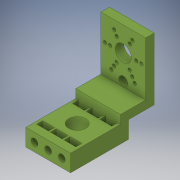
# Autodesk Inventor part: 000.406 - Проставка
Saved by Autodesk Inventor 2019 (Build 230136000, 136)
## iProperties
Created: 2020-02-29
Part Number: 000.406 - Проставка
Material: Пластик АБС
Document SubType Name: Modeling
Designer: Петров Иван
Density: 1.06 g/cm^3
Appearance: Оливково-зеленый
Author: Петров Иван
Autodesk Inventor part; units mm, degrees
ref_plane "YZ Plane" through (0, 0, 0) normal (1, 0, 0) x (0, 1, 0)
ref_plane "XZ Plane" through (0, 0, 0) normal (0, 1, 0) x (-1, 0, 0)
ref_plane "XY Plane" through (0, 0, 0) normal (0, 0, 1) x (1, 0, 0)
sketch "Эскиз1" plane through (0, 0, 0) normal (0, 1, 0) x (-1, 0, 0)
  line L0 (-13.1, 17) -> (13.1, 17)
  line L1 (13.1, 17) -> (13.1, -17)
  line L2 (13.1, -17) -> (-13.1, -17)
  line L3 (-13.1, -17) -> (-13.1, 17)
  line L4 (-13.1, 17) -> (13.1, -17) construction
  line L5 (13.1, 17) -> (-13.1, -17) construction
  point P0 (0, 0)
  dimension "d0" = 26.2
  dimension "d1" = 34
  constraints: 12 end point, 2 midpoint, 2 parallel, 1 horizontal, 1 perpendicular
  measures "d0" distance of L1.end L2.end
  measures "d1" distance of L0.end L1.end
extrude "Выдавливание1" add sketch "Эскиз1" along normal blind 10
sketch "Эскиз2" plane through (-13.1, 0, 17) normal (0, 0, 1) x (1, 0, 0)
  line L0 (0, 10) -> (26.2, 10) projected
  line L1 (13.1, 10) -> (13.1, 5)
  circle A0 centre (13.1, 5) radius 2
  point P0 (13.1, 0)
  dimension "d4" = 5
  dimension "d5" = 4
  constraints: 2 end point, 1 centre point, 1 coincident, 1 midpoint, 1 vertical
  measures "d4" distance of L1.start L1.end
  measures "d5" diameter of A0
extrude "Выдавливание2" cut sketch "Эскиз2" against normal blind 10
sketch "Эскиз4" plane through (0, 10, 0) normal (0, 1, 0) x (1, 0, 0)
  line L0 (2, -7) -> (-2, -7) projected
  line L1 (3.4971, -12.25) -> (-3.4971, -12.25)
  line L2 (-3.4971, -12.25) -> (-3.4971, -8.75)
  line L3 (-3.4971, -8.75) -> (3.4971, -8.75)
  line L4 (3.4971, -8.75) -> (3.4971, -12.25)
  line L5 (3.4971, -12.25) -> (-3.4971, -8.75) construction
  line L6 (-3.4971, -12.25) -> (3.4971, -8.75) construction
  point P0 (0, 0)
  point P1 (0, -10.5)
  dimension "d55" = 10.5
  constraints: 12 end point, 2 midpoint, 2 parallel, 1 perpendicular
  measures "d55" distance of point (0, 0) point (0, -10.5)
extrude "Выдавливание3" cut sketch "Эскиз4" against normal through all
pattern_linear "Прямоуг.массив2" count 3 spacing 8 along (1, 0, 0) of "Выдавливание2", "Выдавливание3" first direction both ways yes
mirror "Зеркальное отражение2" about plane through (0, 0, 0) normal (0, 0, 1) of "Выдавливание2", "Выдавливание3", "Прямоуг.массив2"
sketch "Эскиз5" plane through (0, 10, 0) normal (0, 1, 0) x (1, 0, 0)
  line L0 (-13.1, -17) -> (-13.1, 17) projected
  line L1 (13.1, 17) -> (13.1, -17) projected
  line L2 (-13.1, 17) -> (13.1, 17)
  line L3 (13.1, 17) -> (13.1, 12.25)
  line L4 (13.1, 12.25) -> (-13.1, 12.25)
  line L5 (-13.1, 12.25) -> (-13.1, 17)
  line L6 (-2, 12.25) -> (2, 12.25) projected
  point P0 (0, 0)
  dimension "d17" = 0
  constraints: 8 end point, 2 parallel, 1 horizontal, 1 perpendicular, 1 point on line
  measures "d17" distance between parallel lines of L6 L4
extrude "Выдавливание4" add sketch "Эскиз5" along normal blind 5
sketch "Эскиз7" plane through (13.1, 0, -17) normal (0, 0, -1) x (-1, 0, 0)
  line L0 (26.2, 0) -> (26.2, 15) projected
  line L1 (26.2, 10) -> (0, 10) projected
  line L2 (26.2, 15) -> (0, 15)
  line L3 (0, 15) -> (0, 10)
  line L4 (0, 10) -> (26.2, 10)
  line L5 (26.2, 10) -> (26.2, 15)
  point P0 (13.1, 0)
  constraints: 8 end point, 2 parallel, 1 horizontal, 1 perpendicular
extrude "Выдавливание6" add sketch "Эскиз7" along normal blind 15
sketch "Эскиз8" plane through (0, 15, 0) normal (0, 1, 0) x (1, 0, 0)
  line L0 (-13.1, 32) -> (13.1, 32)
  line L1 (13.1, 32) -> (13.1, 27)
  line L2 (13.1, 27) -> (-13.1, 27)
  line L3 (-13.1, 27) -> (-13.1, 32)
  line L4 (-13.1, 32) -> (13.1, 32) projected
  point P0 (0, 0)
  point P1 (-13.1, 17)
  dimension "d33" = 5
  dimension "d37" = 0
  constraints: 8 end point, 2 parallel, 1 horizontal, 1 perpendicular
  measures "d33" distance of L0.end L1.end
  measures "d37" distance between parallel lines of L4 L0
extrude "Выдавливание7" add sketch "Эскиз8" along normal blind 31.5
sketch "Эскиз10" plane through (-13.1, 15, -27) normal (0, 0, 1) x (1, 0, 0)
  line L0 (0, 0) -> (26.2, 0) projected
  arc A0 (4.1835, 6.1603) -> (7.4622, 3.7057) centre (6.1878, 5.4205) ccw
  line L1 (7.4622, 3.7057) -> (12.988, 10.2609)
  line L2 (12.988, 10.2609) -> (18.2196, 3.9682)
  arc A1 (18.2196, 3.9682) -> (21.9847, 5.5803) centre (19.8625, 5.334) ccw
  line L3 (21.9847, 5.5803) -> (19.0707, 13.6434)
  line L4 (19.0707, 13.6434) -> (27.1362, 15.0277)
  arc A2 (27.1362, 15.0277) -> (27.6225, 19.0945) centre (26.7747, 17.1334) ccw
  line L5 (27.6225, 19.0945) -> (19.1827, 20.6024)
  line L6 (19.1827, 20.6024) -> (22.0165, 28.2795)
  arc A3 (22.0165, 28.2795) -> (18.7378, 30.7341) centre (20.0122, 29.0193) ccw
  line L7 (18.7378, 30.7341) -> (13.212, 24.1789)
  line L8 (13.212, 24.1789) -> (7.9804, 30.4716)
  arc A4 (7.9804, 30.4716) -> (4.2153, 28.8595) centre (6.3375, 29.1058) ccw
  line L9 (4.2153, 28.8595) -> (7.1293, 20.7964)
  line L10 (7.1293, 20.7964) -> (-0.9362, 19.412)
  arc A5 (-0.9362, 19.412) -> (-1.4225, 15.3453) centre (-0.5747, 17.3063) ccw
  line L11 (-1.4225, 15.3453) -> (7.0173, 13.8374)
  line L12 (7.0173, 13.8374) -> (4.1835, 6.1603)
  circle A6 centre (9.2206, 10.5975) radius 1
  circle A7 centre (6.1878, 5.4205) radius 1
  circle A8 centre (2.4252, 17.2874) radius 1
  circle A9 centre (9.3046, 23.8908) radius 1
  circle A10 centre (6.3375, 29.1058) radius 1
  circle A11 centre (18.4958, 26.4308) radius 1
  circle A12 centre (20.7748, 17.1714) radius 1
  circle A13 centre (26.7747, 17.1334) radius 1
  circle A14 centre (18.3789, 7.9415) radius 1
  circle A15 centre (13.1, 17.2199) radius 4.75
  circle A16 centre (19.8625, 5.334) radius 1
  circle A17 centre (16.8954, 10.549) radius 1
  circle A18 centre (23.7748, 17.1524) radius 1
  circle A19 centre (20.0122, 29.0193) radius 1
  circle A20 centre (16.9794, 23.8422) radius 1
  circle A21 centre (7.8211, 26.4983) radius 1
  circle A22 centre (-0.5747, 17.3063) radius 1
  circle A23 centre (5.4252, 17.2684) radius 1
  circle A24 centre (7.7042, 8.009) radius 1
  circle A25 centre (13.1, 17.2199) radius 1.875
  point P0 (13.1, -15)
  dimension "d41" = 6.9599
  dimension "d42" = 6.9599
  dimension "d43" = 6.959
  dimension "d44" = 6.959
  dimension "d45" = 6.9599
  dimension "d46" = 6.9599
  dimension "d47" = 3
  constraints: 26 centre point, 24 end point, 12 point on circle
  measures "d41" distance of L3.end L1.end
  measures "d42" distance of L5.end L7.end
  measures "d43" vertical distance of L3.end L5.end
  measures "d44" vertical distance of L11.end L9.end
  measures "d45" distance of L1.end L11.end
  measures "d46" distance of L7.end L9.end
  measures "d47" distance of A11.centre A20.centre
extrude "Выдавливание9" cut sketch "Эскиз10" against normal blind 34 contours A6 | A7 | A8 | A9 | A11 | A12 | A14 | A15 | A16 | A17 | A18 | A20 | A21 | A23 | A24 | A25
sketch "Эскиз11" plane through (-13.1, 15, -27) normal (0, 0, 1) x (1, 0, 0)
  line L0 (0, 0) -> (26.2, 0) projected
  line L1 (13.1, 0) -> (13.1, 3)
  circle A0 centre (13.1, 3) radius 2.6
  point P0 (13.1, -15)
  dimension "d48" = 3
  dimension "d49" = 5.2
  constraints: 2 end point, 1 centre point, 1 coincident, 1 midpoint, 1 vertical
  measures "d48" distance of L1.start L1.end
  measures "d49" diameter of A0
extrude "Выдавливание10" cut sketch "Эскиз11" against normal blind 42.5
sketch "Эскиз12" plane through (0, 10, 0) normal (0, 1, 0) x (1, 0, 0)
  circle A0 centre (0, 0) radius 5
  dimension "d52" = 10
  constraints: 1 centre point, 1 coincident
  measures "d52" diameter of A0
extrude "Выдавливание11" cut sketch "Эскиз12" against normal blind 10
